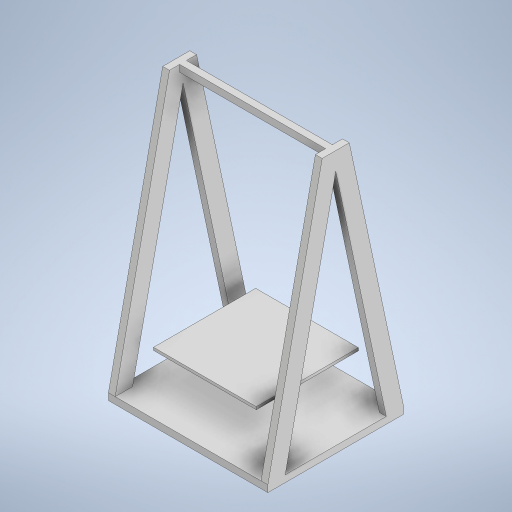
# Autodesk Inventor part: Estructura AA
Saved by Autodesk Inventor 2024 (Build 280153000, 153)
## iProperties
Created: 2024-07-20
Part Number: Estructura AA
Material: Generic
Document SubType Name: Modeling
Designer: compu
Density: 1 g/cm^3
Appearance: Default
Author: compu
Autodesk Inventor part; units mm, degrees
ref_plane "YZ Plane" through (0, 0, 0) normal (1, 0, 0) x (0, 1, 0)
ref_plane "XZ Plane" through (0, 0, 0) normal (0, 1, 0) x (-1, 0, 0)
sketch "Sketch1" plane through (0, 0, 0) normal (0, 1, 0) x (-1, 0, 0)
  line L0 (235, -200) -> (-235, -200)
  line L1 (-235, -200) -> (-235, 200)
  line L2 (-235, 200) -> (235, 200)
  line L3 (235, 200) -> (235, -200)
  line L4 (329, 0) -> (-329, 0) projected
  line L5 (0, -280) -> (0, 280) projected
  point P0 (0, 0)
  dimension "d0" = 470
  dimension "d1" = 400
  constraints: 8 end point, 2 parallel, 1 horizontal, 1 perpendicular, 2 other
  measures "d0" distance of L0.start L0.end
  measures "d1" distance of L0.end L1.end
extrude "Extrusion1" add sketch "Sketch1" along normal blind 20
sketch "Sketch2" plane through (0, 20, 0) normal (0, 1, 0) x (1, 0, 0)
  line L0 (-235, -200) -> (235, -200) projected
  line L1 (235, -200) -> (235, 200) projected
  line L2 (235, 200) -> (-235, 200) projected
  line L3 (-235, 200) -> (-235, -200) projected
  line L4 (-329, 0) -> (329, 0) projected
  line L5 (0, 280) -> (0, -280) projected
  circle A0 centre (0, 0) radius 20
  dimension "d4" = 40
  constraints: 1 centre point, 1 coincident
  measures "d4" diameter of A0
extrude "Extrusion2" add sketch "Sketch2" along normal blind 125 contours A0 L4 L5 | L5 L4 A0 | A0 L5 L4 | L5 A0 L4
sketch "Sketch3" plane through (0, 145, 0) normal (0, 1, 0) x (1, 0, 0)
  line L0 (-151.5, 150.5) -> (151.5, 150.5)
  line L1 (151.5, 150.5) -> (151.5, -150.5)
  line L2 (151.5, -150.5) -> (-151.5, -150.5)
  line L3 (-151.5, -150.5) -> (-151.5, 150.5)
  line L4 (-329, 0) -> (329, 0) projected
  line L5 (0, 280) -> (0, -280) projected
  point P0 (0, 0)
  dimension "d7" = 303
  dimension "d8" = 301
  constraints: 8 end point, 2 parallel, 1 horizontal, 1 perpendicular, 2 other
  measures "d7" distance of L1.end L2.end
  measures "d8" distance of L0.end L1.end
extrude "Extrusion3" add sketch "Sketch3" along normal blind 8
ref_plane "Work Plane1" through (0, 753, 0) normal (0, 1, 0) x (1, 0, 0)
sketch "Sketch4" plane through (0, 753, 0) normal (0, 1, 0) x (1, 0, 0)
  line L0 (-235, 10) -> (235, 10)
  line L1 (235, 10) -> (235, -10)
  line L2 (235, -10) -> (-235, -10)
  line L3 (-235, -10) -> (-235, 10)
  circle A0 centre (0, 0) radius 20 projected
  line L4 (-235, -200) -> (235, -200) projected
  line L5 (235, -200) -> (235, 200) projected
  line L6 (235, 200) -> (-235, 200) projected
  line L7 (-235, 200) -> (-235, -200) projected
  line L8 (-329, 0) -> (329, 0) projected
  line L9 (0, 280) -> (0, -280) projected
  dimension "d12" = 20
  constraints: 8 end point, 2 collinear, 2 parallel, 1 horizontal, 1 perpendicular, 1 other
  measures "d12" distance of L0.end L1.end
extrude "Extrusion4" add sketch "Sketch4" along normal blind 20 contours L0 A0 L8 L3 | L0 L9 L8 A0 | L8 A0 L2 L3 | L0 A0 L8 L9 | L8 L9 L2 A0 | L0 L1 L8 A0 | L8 A0 L2 L9 | L8 L1 L2 A0
sketch "Sketch5" plane through (235, 0, 200) normal (1, 0, 0) x (0, 0, -1)
  line L0 (190, 753) -> (210, 753) projected
  line L1 (210, 753) -> (210, 773) projected
  line L2 (190, 773) -> (210, 773) projected
  line L3 (190, 753) -> (190, 773) projected
  line L4 (0, 0) -> (400, 0) projected
  line L5 (0, 20) -> (400, 20) projected
  line L6 (0, 0) -> (0, 20) projected
  line L7 (400, 0) -> (400, 20) projected
  line L8 (0, 0) -> (400, 0) projected
  line L9 (400, 0) -> (400, 20) projected
  line L10 (0, 20) -> (400, 20) projected
  line L11 (0, 0) -> (0, 20) projected
  line L12 (160.0551, 773) -> (239.9449, 773)
  line L13 (0, 20) -> (160.0551, 773)
  line L14 (200, -184.6) -> (200, 1107.6) projected
  line L15 (400, 20) -> (239.9449, 773)
  line L16 (190, 773) -> (210, 773) projected
  line L17 (0, 20) -> (51.117, 20)
  line L18 (348.883, 20) -> (400, 20)
  line L19 (348.883, 20) -> (200, 720.4393)
  line L20 (51.117, 20) -> (200, 720.4393)
  line L21 (150, 690) -> (250, 690) construction
  line L22 (250, 690) -> (250, 563) construction
  line L23 (250, 563) -> (150, 563) construction
  line L24 (150, 563) -> (150, 690) construction
  point P0 (200, 0)
  point P1 (183.5455, 773)
  point P2 (216.4545, 773)
  dimension "d16" = 78
  dimension "d18" = 78
  dimension "d26" = 50
  dimension "d27" = 100
  dimension "d28" = 127
  dimension "d29" = 670
  constraints: 22 end point, 4 parallel, 3 collinear, 2 horizontal, 2 point on line, 2 symmetric about line, 1 perpendicular, 1 other
  measures "d16" angle of L5 L13
  measures "d18" angle of L5 L15
  measures "d26" distance between parallel lines of L20 L13
  measures "d27" distance of L21.start L21.end
  measures "d28" distance of L21.end L22.end
  measures "d29" distance between parallel lines of L5 L21
extrude "Extrusion5" add sketch "Sketch5" against normal blind 20 contours L3 L2 L14 L0 | L0 L14 L20 L5 L13 L12 L3 | L14 L2 L1 L0 | L0 L1 L12 L15 L5 L19 L14
sketch "Sketch6" plane through (-235, 753, -10) normal (-1, 0, 0) x (0, 0, 1)
  line L0 (-40, -60) -> (60, -60) construction
  line L1 (60, -60) -> (60, -188) construction
  line L2 (60, -188) -> (-40, -188) construction
  line L3 (-40, -188) -> (-40, -60) construction
  line L4 (10, -925.1189) -> (10, 279.7131) projected
  line L5 (0, 0) -> (20, 0) projected
  line L6 (20, 0) -> (20, 20) projected
  line L7 (0, 20) -> (20, 20) projected
  line L8 (0, 0) -> (0, 20) projected
  line L9 (20, 0) -> (20, 20) projected
  line L10 (0, 0) -> (20, 0) projected
  line L11 (0, 20) -> (0, 0) projected
  line L12 (0, 20) -> (-29.9449, 20) projected
  line L13 (-29.9449, 20) -> (-190, -733) projected
  line L14 (-138.883, -733) -> (-190, -733) projected
  line L15 (210, -733) -> (49.9449, 20) projected
  line L16 (49.9449, 20) -> (20, 20) projected
  line L17 (-29.9449, 20) -> (-190, -733) projected
  line L18 (-190, -733) -> (-29.9449, 20)
  line L19 (-29.9449, 20) -> (49.9449, 20)
  line L20 (210, -733) -> (49.9449, 20)
  line L21 (159.2287, -733) -> (210, -733)
  line L22 (159.2287, -733) -> (39.7909, 107.5943)
  line L23 (-138.883, -733) -> (39.7909, 107.5943) projected
  line L24 (39.7909, 107.5943) -> (-138.883, -733)
  line L25 (-138.883, -733) -> (-190, -733)
  line L26 (-138.883, -733) -> (10, -32.5607) projected
  line L27 (10, -32.5607) -> (158.883, -733) projected
  line L28 (210, -733) -> (158.883, -733) projected
  point P0 (10, -753)
  point P1 (0, 20)
  dimension "d21" = 100
  dimension "d22" = 128
  dimension "d23" = 60
  constraints: 22 end point, 4 collinear, 2 horizontal, 2 parallel, 1 perpendicular, 1 other
  measures "d21" distance of L0.start L0.end
  measures "d22" distance of L0.end L1.end
  measures "d23" distance between parallel lines of L5 L0
extrude "Extrusion6" add sketch "Sketch6" against normal blind 20 contours L23 L14 L13 L12 L8 L5 L4 | L4 L5 L23 | L23 L5 L6 L16 L15 L22 L28 L27 | L6 L16 L23 | L22 L15 L21
body "Solid1"
